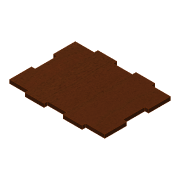
# Autodesk Inventor part: M06 - Wall Side 1
Saved by Autodesk Inventor 2016 (Build 200138000, 138)
## iProperties
Created: 2016-12-26
Part Number: M06 - Wall Side 1
Material: Wood (Walnut)
Document SubType Name: Modeling
Designer: Fernando
Stock Number: 0
Mass: 136.491 g
Surface Area: 684.893 cm^2
Volume: 248.165 cm^3
Density: 0.55 g/cm^3
Appearance: Walnut - Natural Polished
SurfaceArea_m2: .07
Author: Fernando
Autodesk Inventor part; units mm, degrees
ref_plane "YZ Plane" through (0, 0, 0) normal (1, 0, 0) x (0, 1, 0)
ref_plane "XZ Plane" through (0, 0, 0) normal (0, 1, 0) x (-1, 0, 0)
ref_plane "XY Plane" through (0, 0, 0) normal (0, 0, 1) x (1, 0, 0)
sketch "Sketch2" plane through (0, 0, 0) normal (0, 0, 1) x (1, 0, 0)
  line L0 (-105, -72.5) -> (105, -72.5)
  line L1 (105, -72.5) -> (105, 72.5)
  line L2 (105, 72.5) -> (-105, 72.5)
  line L3 (-105, 72.5) -> (-105, -72.5)
  line L4 (-105, -72.5) -> (105, 72.5) construction
  line L5 (105, -72.5) -> (-105, 72.5) construction
  point P0 (0, 0)
  dimension "d11" = 145
  dimension "d12" = 210
  constraints: 12 end point, 2 midpoint, 2 parallel, 1 horizontal, 1 perpendicular
  measures "d11" distance of L2.end L0.start
  measures "d12" distance of L1.end L2.end
extrude "Extrusion2" add sketch "Sketch2" along normal blind 8
sketch "Sketch3" plane through (0, 0, 8) normal (0, 0, 1) x (1, 0, 0)
  line L0 (105, 72.5) -> (-105, 72.5) projected
  line L1 (-63, 72.5) -> (-21, 72.5)
  line L2 (-21, 72.5) -> (-21, 80.5)
  line L3 (-21, 80.5) -> (-63, 80.5)
  line L4 (-63, 80.5) -> (-63, 72.5)
  line L5 (63, 72.5) -> (21, 72.5)
  line L6 (21, 72.5) -> (21, 80.5)
  line L7 (21, 80.5) -> (63, 80.5)
  line L8 (63, 80.5) -> (63, 72.5)
  line L9 (-21, 80.5) -> (21, 80.5) construction
  line L10 (63, 80.5) -> (105, 80.5) construction
  line L11 (-63, 80.5) -> (-105, 80.5) construction
  point P0 (0, 0)
  dimension "d15" = 8
  constraints: 22 end point, 4 collinear, 4 horizontal, 4 parallel, 4 point on line, 2 perpendicular, 2 vertical alignment
  measures "d15" distance of L3.end L1.start
extrude "Extrusion3" add sketch "Sketch3" against normal blind 8
mirror "Mirror1" about plane through (0, 0, 0) normal (0, 1, 0) of "Extrusion3"
sketch "Sketch4" plane through (0, 0, 8) normal (0, 0, 1) x (1, 0, 0)
  line L0 (-105, 72.5) -> (-105, -72.5) projected
  line L1 (-105, 24.1667) -> (-97, 24.1667)
  line L2 (-97, 24.1667) -> (-97, -24.1667)
  line L3 (-97, -24.1667) -> (-105, -24.1667)
  line L4 (-105, -24.1667) -> (-105, 24.1667)
  line L5 (-97, 24.1667) -> (-97, 72.5) construction
  line L6 (-97, -24.1667) -> (-97, -72.5) construction
  point P0 (0, 0)
  dimension "d20" = 8
  constraints: 12 end point, 2 collinear, 2 horizontal alignment, 2 parallel, 2 vertical, 1 horizontal, 1 perpendicular, 1 point on line
  measures "d20" distance between parallel lines of L0 L2
extrude "Extrusion4" cut sketch "Sketch4" against normal blind 8
mirror "Mirror2" about plane through (0, 0, 0) normal (1, 0, 0) of "Extrusion4"
body "Solid2"
